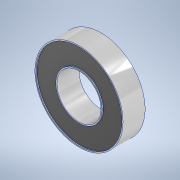
# Autodesk Inventor part: bearing
Saved by Autodesk Inventor 2020.1 (Build 241239000, 239)
## iProperties
Created: 2019-11-19
Part Number: bearing
Material: Aluminum 6061
Document SubType Name: Modeling
Designer: 19Bar
Density: 2.7 g/cm^3
Appearance: Aluminum - Flat
Author: 19Bar
Autodesk Inventor part; units mm, degrees
ref_plane "YZ Plane" through (0, 0, 0) normal (1, 0, 0) x (0, 1, 0)
ref_plane "XZ Plane" through (0, 0, 0) normal (0, 1, 0) x (-1, 0, 0)
ref_plane "XY Plane" through (0, 0, 0) normal (0, 0, 1) x (1, 0, 0)
sketch "Sketch1" plane through (0, 0, 0) normal (0, 0, 1) x (1, 0, 0)
  circle A0 centre (0, 0) radius 5
  circle A1 centre (0, 0) radius 10
  dimension "d0" = 10
  dimension "d1" = 20
  constraints: 2 centre point, 2 coincident
  measures "d0" diameter of A0
  measures "d1" diameter of A1
extrude "Extrusion1" add sketch "Sketch1" along normal blind 4.5
sketch "Sketch2" plane through (0, 0, 4.5) normal (0, 0, 1) x (1, 0, 0)
  circle A0 centre (0, 0) radius 10
  circle A1 centre (0, 0) radius 9.75
  circle A2 centre (0, 0) radius 5
  circle A3 centre (0, 0) radius 5.25
  dimension "d4" = 19.5
  dimension "d5" = 10
  dimension "d6" = 10.5
  constraints: 4 centre point, 4 coincident
  measures "d4" diameter of A1
  measures "d5" diameter of A2
  measures "d6" diameter of A3
extrude "Extrusion2" add sketch "Sketch2" along normal blind 0.25
sketch "Sketch3" plane through (0, 0, 0) normal (0, 0, -1) x (-1, 0, 0)
  circle A0 centre (0, 0) radius 10
  circle A1 centre (0, 0) radius 9.75
  circle A2 centre (0, 0) radius 5
  circle A3 centre (0, 0) radius 5.25
  dimension "d9" = 20
  dimension "d10" = 19.5
  dimension "d11" = 10
  dimension "d12" = 10.5
  constraints: 4 centre point, 4 coincident
  measures "d9" diameter of A0
  measures "d10" diameter of A1
  measures "d11" diameter of A2
  measures "d12" diameter of A3
extrude "Extrusion3" add sketch "Sketch3" along normal blind 0.25
body "Solid1"
